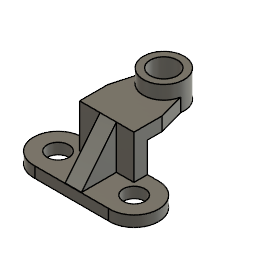
Record 4 (Autodesk Fusion 360 design; units mm, degrees)
part number: 2026-02-17-13-34-41-217
Autodesk Fusion 360 part; units mm, degrees
note: some values were not read from the file. Set by a fixed rule: which sketch regions a step uses.
sketch "Sketch1" plane through (0, 0, 0) normal (0, 1, 0) x (1, 0, 0)
  circle A0 centre (-29.052, 0) radius 8
  circle A1 centre (26.948, 0) radius 8
  line L0 (-29, -17.9738) -> (27, -17.9738)
  line L1 (-29, 17.9738) -> (27, 17.9738)
  arc A2 (25.9777, -17.9738) -> (25.9777, 17.9738) centre (26.948, 0) ccw
  arc A3 (-28.0816, 17.9738) -> (-28.0816, -17.9738) centre (-29.052, 0) ccw
  dimension "d1" = 56
  dimension "d2" = 16
  dimension "d3" = 16
  dimension "d5" = 36
  dimension "d6" = 36
  constraint horizontal L0
  constraint concentric A0 A3
  constraint concentric A1 A2
  constraint coincident L0 A2.start
  constraint coincident L1 A2.end
  constraint coincident L1 A3.start
  constraint coincident L0 A3.end
  measures "d1" distance of A0.centre A1.centre
  measures "d2" diameter of A0
  measures "d3" diameter of A1
  measures "d5" diameter of A3
  measures "d6" diameter of A2
extrude "Extrude1" add sketch "Sketch1" along normal blind 8
sketch "Sketch2" plane through (0, 8, 0) normal (0, 1, 0) x (-1, 0, 0)
  circle A0 centre (-26.948, 0) radius 8
  circle A1 centre (29.052, 0) radius 8
  arc A2 (28.0816, -17.9738) -> (28.0816, 17.9738) centre (29.052, 0) ccw
  line L0 (28.0816, 17.9738) -> (-25.9777, 17.9738)
  arc A3 (-25.9777, 17.9738) -> (-25.9777, -17.9738) centre (-26.948, 0) ccw
  line L1 (-25.9777, -17.9738) -> (28.0816, -17.9738)
  line L2 (21.1928, -17.9738) -> (-18.8072, -17.9738)
  line L3 (-18.8072, -17.9738) -> (-18.8072, -7.9738)
  line L4 (-18.8072, -7.9738) -> (21.1928, -7.9738)
  line L5 (21.1928, -7.9738) -> (21.1928, -17.9738)
  dimension "d9" = 40
  dimension "d10" = 10
  dimension "d11" = 40
  dimension "d12" = 40
  dimension "d13" = 10
  constraint horizontal L2
  constraint vertical L3
  constraint horizontal L4
  constraint vertical L5
  constraint coincident L1 L2.start
  measures "d9" distance of L3.end L4.end
  measures "d10" distance of L2.start L4.end
  measures "d11" distance of L3.end L4.end
  measures "d12" distance of L3.end L4.end
  measures "d13" distance of L2.end L3.end
extrude "Extrude2" add sketch "Sketch2" along normal blind 32 contours L1 L2 L3 L4 L5
sketch "Sketch3" plane through (0, 0, -17.9738) normal (0, 0, -1) x (-1, 0, 0)
  line L0 (-25.9777, 0) -> (28.0816, 0)
  line L1 (28.0816, 0) -> (28.0816, 8)
  line L2 (28.0816, 8) -> (21.1928, 8)
  line L3 (21.1928, 8) -> (21.1928, 40)
  line L4 (21.1928, 40) -> (-18.8072, 40)
  line L5 (-18.8072, 40) -> (-18.8072, 8)
  line L6 (-18.8072, 8) -> (-25.9777, 8)
  line L7 (-25.9777, 8) -> (-25.9777, 0)
  line L8 (-18.8072, 40) -> (21.1928, 40)
  line L9 (21.1928, 40) -> (21.1928, 30)
  line L10 (21.1928, 30) -> (-18.8072, 30)
  line L11 (-18.8072, 30) -> (-18.8072, 40)
  dimension "d16" = 10
  constraint horizontal L8
  constraint vertical L9
  constraint horizontal L10
  constraint vertical L11
  constraint coincident L3 L9.end
  constraint coincident L4.end L5.start
  measures "d16" distance of L4.end L10.end
extrude "Extrude3" add sketch "Sketch3" along normal blind 32 contours L3 L4 L5 L8 L9 L10 L11
sketch "Sketch4" plane through (0, 40, 0) normal (0, 1, 0) x (-1, 0, 0)
  line L0 (21.1928, -7.9738) -> (-18.8072, -7.9738)
  line L1 (-18.8072, -7.9738) -> (-18.8072, -49.9738)
  line L2 (-18.8072, -49.9738) -> (21.1928, -49.9738)
  line L3 (21.1928, -49.9738) -> (21.1928, -7.9738)
  line L4 (21.1928, -28.6563) -> (15.1408, -50.6921)
  line L5 (-19.0097, -28.6563) -> (-12.9578, -50.6921)
  constraint coincident L3 L4.start
extrude "Extrude4" cut sketch "Sketch4" against normal blind 20 contours L2 L3 L4
sketch "Sketch5" plane through (0, 40, 0) normal (0, 1, 0) x (-1, 0, 0)
  line L0 (15.3381, -49.9738) -> (21.1928, -28.6563)
  line L1 (21.1928, -28.6563) -> (21.1928, -7.9738)
  line L2 (21.1928, -7.9738) -> (-18.8072, -7.9738)
  line L3 (-18.8072, -7.9738) -> (-18.8072, -49.9738)
  line L4 (-18.8072, -49.9738) -> (15.3381, -49.9738)
  line L5 (1.1928, 40.1018) -> (1.1928, -51.5866)
  line L6 (-12.9526, -49.9738) -> (-18.8072, -28.6563)
  constraint perpendicular L4 L5
  constraint symmetric L0.start L5 L6.start
  constraint symmetric L0.end L5 L6.end
extrude "Extrude5" cut sketch "Sketch5" against normal blind 30 contours L3 L4 L6
sketch "Sketch6" plane through (0, 40, 0) normal (0, 1, 0) x (-1, 0, 0)
  line L0 (-18.8072, -28.6563) -> (-12.9526, -49.9738)
  line L1 (-12.9526, -49.9738) -> (15.3381, -49.9738)
  line L2 (15.3381, -49.9738) -> (21.1928, -28.6563)
  line L3 (21.1928, -28.6563) -> (21.1928, -7.9738)
  line L4 (21.1928, -7.9738) -> (-18.8072, -7.9738)
  line L5 (-18.8072, -7.9738) -> (-18.8072, -28.6563)
  circle A0 centre (1.1928, -49.9738) radius 15
  circle A1 centre (1.1928, -49.9738) radius 10
  dimension "d23" = 30
  dimension "d24" = 20
  constraint midpoint L1 A0.centre
  constraint concentric A0 A1
  measures "d23" diameter of A0
  measures "d24" diameter of A1
extrude "Extrude6" add sketch "Sketch6" along normal blind 10 contours L0 L1 L2 A0 A1 | L0 L1 L2 A0 A1
extrude "Extrude7" add 1 faces at (1.7657, 40, -62.9484) along direction (0, -1, 0) blind 10
extrude "Extrude8" cut 1 faces at (-2.2646, 40, -45.2778) along direction (0, -1, 0) blind 45
sketch "Sketch7" plane through (0, 8, 0) normal (0, 1, 0) x (-1, 0, 0)
  line L0 (-18.8072, -17.9738) -> (-18.8072, -7.9738)
  line L1 (-18.8072, -7.9738) -> (21.1928, -7.9738)
  line L2 (21.1928, -7.9738) -> (21.1928, -17.9738)
  line L3 (21.1928, -17.9738) -> (28.0816, -17.9738)
  arc A0 (28.0816, -17.9738) -> (28.0816, 17.9738) centre (29.052, 0) ccw
  line L4 (28.0816, 17.9738) -> (-25.9777, 17.9738)
  arc A1 (-25.9777, 17.9738) -> (-25.9777, -17.9738) centre (-26.948, 0) ccw
  line L5 (-25.9777, -17.9738) -> (-18.8072, -17.9738)
  circle A2 centre (29.052, 0) radius 8
  circle A3 centre (-26.948, 0) radius 8
  line L6 (6.0956, -7.9738) -> (-5.9044, -7.9738)
  line L7 (-5.9044, -7.9738) -> (-5.9044, 17.6922)
  line L8 (-5.9044, 17.6922) -> (6.0956, 17.6922)
  line L9 (6.0956, 17.6922) -> (6.0956, -7.9738)
  dimension "d31" = 12
  constraint horizontal L6
  constraint vertical L7
  constraint horizontal L8
  constraint vertical L9
  constraint coincident L1 L6.start
  measures "d31" distance of L6.start L6.end
extrude "Extrude9" add sketch "Sketch7" along normal blind 32 contours L1 L6 L7 L8 L9
sketch "Sketch8" plane through (5.9044, 0, 0) normal (1, 0, 0) x (0, 0, -1)
  line L0 (-17.6922, 8) -> (7.9738, 8)
  line L1 (7.9738, 8) -> (7.9738, 40)
  line L2 (7.9738, 40) -> (-17.6922, 40)
  line L3 (-17.6922, 40) -> (-17.6922, 8)
  line L4 (-17.6922, 8) -> (7.9738, 40)
  constraint coincident L0.start L3.end
  constraint coincident L1.end L2.start
extrude "Extrude10" cut sketch "Sketch8" against normal blind 55 contours L2 L3 L4
